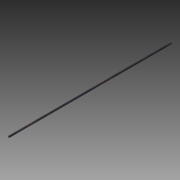
# Autodesk Inventor part: Rudder_Hinge_Pin
Saved by Autodesk Inventor 2011 SP1 (Build 150282100, 282)
## iProperties
Created: 2011-06-11
Part Number: Rudder_Hinge_Pin
Document SubType Name: Modeling
Designer: Andrew G. Meyer
Density: 1 g/cm^3
Mass: 0.866541 g
Surface Area: 15.4117 cm^2
Volume: 0.866541 cm^3
Author: Andrew G. Meyer
Autodesk Inventor part; units mm, degrees
ref_plane "YZ Plane" through (0, 0, 0) normal (1, 0, 0) x (0, 1, 0)
ref_plane "XZ Plane" through (0, 0, 0) normal (0, 1, 0) x (-1, 0, 0)
ref_plane "XY Plane" through (0, 0, 0) normal (0, 0, 1) x (1, 0, 0)
sketch "Sketch1" plane through (0, 0, 0) normal (0, 0, 1) x (1, 0, 0)
  circle A0 centre (0, 0) radius 1.1303
  dimension "d0" = 2.2606
  constraints: 1 centre point, 1 coincident
  measures "d0" diameter of A0
extrude "Extrusion1" add sketch "Sketch1" along normal blind 215.9
fillet "Fillet1" radius 0.0254 2 edges at (-1.1303, 0, 215.9) (-1.1303, 0, 0)
body "Solid1"
